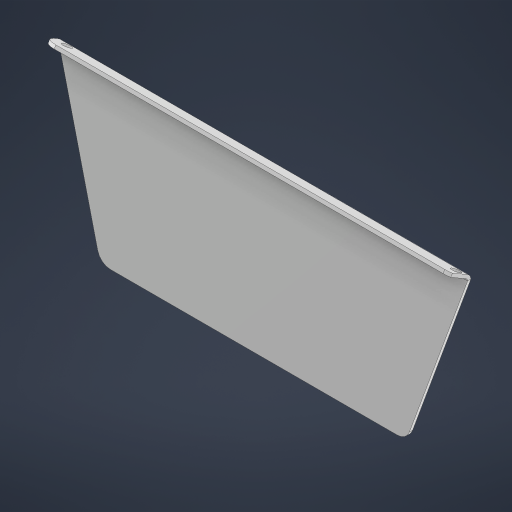
# Autodesk Inventor part: wing_wedge
Saved by Autodesk Inventor 2024 (Build 280153000, 153)
## iProperties
Created: 2024-01-16
Part Number: wing_wedge
Material: Acetal Resin, White
Document SubType Name: Modeling
Designer: avere
Density: 1.425 g/cm^3
Appearance: Smooth - White
Author: avere
Autodesk Inventor part; units mm, degrees
ref_plane "YZ Plane" through (0, 0, 0) normal (1, 0, 0) x (0, 1, 0)
ref_plane "XZ Plane" through (0, 0, 0) normal (0, 1, 0) x (-1, 0, 0)
ref_plane "XY Plane" through (0, 0, 0) normal (0, 0, 1) x (1, 0, 0)
sketch "Sketch1" plane through (0, 0, 0) normal (0, 0, 1) x (1, 0, 0)
  line L0 (26.2341, -88.9) -> (159.0469, -88.9)
  circle A0 centre (190.5233, -0.0123) radius 2.1844
  arc A1 (193.5393, 5.5758) -> (190.4426, 6.3372) centre (190.5233, -0.0123) ccw
  line L1 (165.0634, -0.0075) -> (177.7634, -0.0075) construction
  line L2 (190.4426, 6.3372) -> (182.7263, 6.3372)
  line L3 (182.7263, 6.3372) -> (-0.0289, 6.3363)
  line L4 (193.5393, 5.5758) -> (193.5393, -6.3491)
  line L5 (193.5393, -6.3491) -> (165.014, -84.7218)
  arc A2 (159.0469, -88.9) -> (165.014, -84.7218) centre (159.0469, -82.55) ccw
  circle A3 centre (-0.0565, -0.0137) radius 2.1845
  arc A4 (-0.0289, 6.3363) -> (-6.4066, -0.0138) centre (-0.0565, -0.0137) ccw
  line L6 (26.2341, -88.9) -> (18.6122, -88.9)
  arc A5 (12.4412, -84.0472) -> (18.6122, -88.9) centre (18.6122, -82.55) ccw
  line L7 (193.5393, -6.3491) -> (-6.4065, -6.3491)
  line L8 (-6.4066, -0.0137) -> (-6.4065, -6.3637)
  line L9 (-6.4065, -6.3637) -> (12.4412, -84.0472)
  point P0 (157.3842, 6.3371)
  point P1 (13.5341, -88.9)
  dimension "d9" = 4.3688
  dimension "d26" = 6.35
  dimension "d29" = 12.7
  dimension "d30" = 6.35
  constraints: 20 end point, 9 point on circle, 6 centre point, 4 horizontal, 4 point on line, 4 tangent, 2 coincident
  measures "d9" diameter of A0
  measures "d26" radius of A2
  measures "d29" distance of L0.start point (13.534, -88.9)
  measures "d30" radius of A5
extrude "Extrusion1" add sketch "Sketch1" along normal blind 1.5875
bend part "Bend Part1" radius 3.175 angle 60 line through (193.5393, -6.3491, 0) along (-1, 0, 0) centre toward (0, 0, 1) moving side (0, 1, 0) both sides no
body "Solid1"
